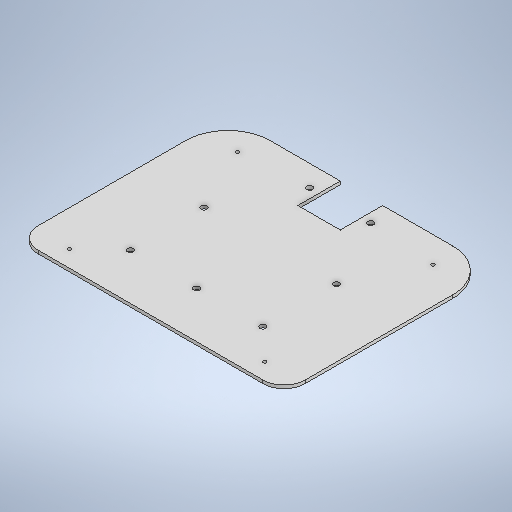
# Autodesk Inventor part: Chassis Rear Plate
Saved by Autodesk Inventor 2025.2 (Build 292293000, 293)
## iProperties
Created: 2025-02-20
Part Number: Chassis Rear Plate
Material: Generic
Document SubType Name: Modeling
Designer: Matt Tidd
Density: 1 g/cm^3
Appearance: Default
Author: Matt Tidd
Autodesk Inventor part; units mm, degrees
ref_plane "YZ Plane" through (0, 0, 0) normal (1, 0, 0) x (0, 1, 0)
ref_plane "XZ Plane" through (0, 0, 0) normal (0, 1, 0) x (-1, 0, 0)
ref_plane "XY Plane" through (0, 0, 0) normal (0, 0, 1) x (1, 0, 0)
sketch "Sketch1" plane through (0, 0, 0) normal (0, 1, 0) x (-1, 0, 0)
  line L0 (126, -23.5) -> (126, 23.5)
  line L1 (126, 23.5) -> (-126, 23.5)
  line L2 (-126, 23.5) -> (-126, -23.5)
  line L3 (82.5, -115.5) -> (82.5, -33.5)
  line L4 (0, 23.5) -> (0, -23.5) construction
  line L5 (-82.5, -115.5) -> (-82.5, -33.5)
  line L6 (42.5, -155.5) -> (-42.5, -155.5)
  line L7 (-126, -23.5) -> (-92.5, -23.5)
  line L8 (92.5, -23.5) -> (126, -23.5)
  arc A0 (-82.5, -33.5) -> (-92.5, -23.5) centre (-92.5, -33.5) ccw
  arc A1 (92.5, -23.5) -> (82.5, -33.5) centre (92.5, -33.5) ccw
  line L9 (0, 23.5) -> (0, -155.5) construction
  line L10 (20, -155.5) -> (-20, -155.5)
  line L11 (-20, -155.5) -> (-20, -115.5)
  line L12 (-20, -115.5) -> (20, -115.5)
  line L13 (20, -115.5) -> (20, -155.5)
  circle A2 centre (0, 0) radius 2.75
  circle A3 centre (62.5, 0) radius 2.75
  circle A4 centre (-62.5, 0) radius 2.75
  circle A5 centre (62.5, -69.5) radius 2.75
  circle A6 centre (-62.5, -69.5) radius 2.75
  circle A7 centre (28.75, -135.5) radius 2.75
  circle A8 centre (-28.75, -135.5) radius 2.75
  line L14 (82.5, -115.5) -> (82.5, -155.5)
  line L15 (82.5, -155.5) -> (42.5, -155.5)
  line L16 (-42.5, -155.5) -> (-82.5, -155.5)
  line L17 (-82.5, -155.5) -> (-82.5, -115.5)
  line L18 (126, -23.5) -> (-126, -23.5)
  line L19 (-126, -23.5) -> (-126, -155.5)
  line L20 (-126, -155.5) -> (126, -155.5)
  line L21 (126, -155.5) -> (126, -23.5)
  line L22 (126, 23.5) -> (-126, 23.5)
  line L23 (-126, 23.5) -> (-126, 43.5)
  line L24 (-126, 43.5) -> (126, 43.5)
  line L25 (126, 43.5) -> (126, 23.5)
  point P0 (82.5, -23.5)
  point P1 (-82.5, -23.5)
  point P2 (0, -135.5)
  dimension "d0" = 252
  dimension "d1" = 47
  dimension "d4" = 10
  dimension "d5" = 40
  dimension "d6" = 40
  dimension "d7" = 5.5
  dimension "d8" = 5.5
  dimension "d9" = 5.5
  dimension "d10" = 5.5
  dimension "d16" = 20
  constraints: 52 end point, 9 centre point, 9 parallel, 7 point on line, 6 horizontal, 6 perpendicular, 6 symmetric about line, 4 point on circle, 4 tangent, 2 coincident, 2 midpoint, 1 collinear, 1 equal radius, 1 vertical, 3 other
  measures "d0" distance of L1.end L0.end
  measures "d1" distance of L0.end L0.start
  measures "d4" radius of A0
  measures "d5" distance of L11.end L12.end
  measures "d6" distance of L10.end L11.end
  measures "d7" diameter of A2
  measures "d8" diameter of A3
  measures "d9" diameter of A5
  measures "d10" diameter of A7
  measures "d16" distance of L22.end L23.end
extrude "Extrusion1" add sketch "Sketch1" along normal blind 3 contours L8 L18 L7 L2 L1 L0 | L21 L20 L14 L3 A1 L8 | L1 L23 L24 L25 | A1 L3 L14 L15 L6 L13 L12 L11 L16 L17 L5 A0 L18 | A0 L5 L17 L20 L19 L7
fillet "Fillet3" radius 40 2 edges at (126, 1.5, -155.5) (-126, 1.5, -155.5)
fillet "Fillet4" radius 20 2 edges at (126, 1.5, 43.5) (-126, 1.5, 43.5)
sketch "Sketch2" plane through (0, 3, 0) normal (0, 1, 0) x (1, 0, 0)
  line L0 (-92.17, 130.7671) -> (92.17, 130.7671) construction
  line L1 (92.17, 130.7671) -> (92.17, -27.8329) construction
  line L2 (92.17, -27.8329) -> (-92.17, -27.8329) construction
  line L3 (-92.17, -27.8329) -> (-92.17, 130.7671) construction
  line L4 (0, 150.8633) -> (0, -88.711) construction
  line L5 (20, 115.5) -> (-20, 115.5) projected
  circle A0 centre (-92.17, 130.7671) radius 1.5
  circle A1 centre (92.17, 130.7671) radius 1.5
  circle A2 centre (-92.17, -27.8329) radius 1.5
  circle A3 centre (92.17, -27.8329) radius 1.5
  point P0 (0, 0)
  point P1 (0, 115.5)
  dimension "d18" = 184.34
  dimension "d19" = 158.6
  dimension "d20" = 3
  constraints: 10 end point, 4 centre point, 4 coincident, 3 equal radius, 2 parallel, 1 horizontal, 1 midpoint, 1 perpendicular, 1 point on line, 1 vertical, 1 other
  measures "d18" distance of L1.end L2.end
  measures "d19" distance of L2.end L0.start
  measures "d20" diameter of A0
extrude "Extrusion2" cut sketch "Sketch2" against normal through all
equation "\"d21\" = d19"
body "Solid1"
